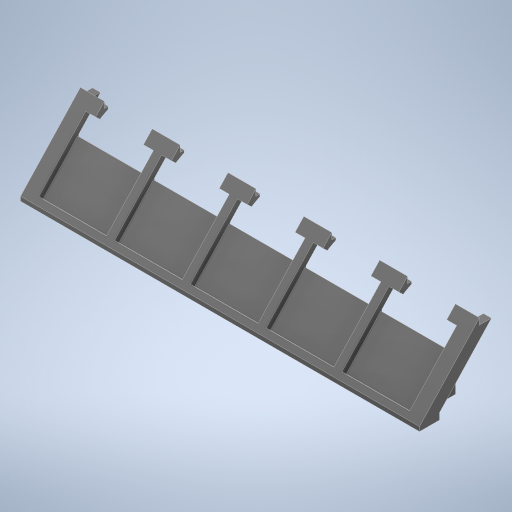
# Autodesk Inventor part: Front
Saved by Autodesk Inventor 2023 (Build 270158000, 158)
## iProperties
Created: 2024-03-20
Part Number: Front
Material: Generic
Document SubType Name: Modeling
Designer: noname
Density: 1 g/cm^3
Appearance: Smooth - Black
Author: noname
Autodesk Inventor part; units mm, degrees
ref_plane "YZ Plane" through (0, 0, 0) normal (1, 0, 0) x (0, 1, 0)
ref_plane "XZ Plane" through (0, 0, 0) normal (0, 1, 0) x (-1, 0, 0)
ref_plane "XY Plane" through (0, 0, 0) normal (0, 0, 1) x (1, 0, 0)
sketch "Sketch1" plane through (0, 0, 0) normal (1, 0, 0) x (0, 1, 0)
  line L0 (0, 0) -> (17.2, -16)
  line L1 (17.2, -16) -> (15.6, -16)
  line L2 (15.6, -16) -> (15.6, -19)
  line L3 (15.6, -19) -> (13.6298, -19)
  line L4 (13.6298, -19) -> (13.6298, -18.142)
  line L5 (1.6, -6) -> (0, -6)
  line L6 (0, -6) -> (0, 0)
  line L7 (1.6, -6) -> (1.6, -6.9515)
  line L8 (1.6, -6.9515) -> (13.6298, -18.142)
  dimension "d0" = 1.6
  dimension "d1" = 1.9702
  dimension "d3" = 14
  dimension "d4" = 4
  dimension "d7" = 6
  dimension "d8" = 3
  dimension "d10" = 10
  dimension "d13" = 1.6
  constraints: 18 end point, 3 perpendicular, 2 parallel, 1 horizontal, 1 vertical
  measures "d0" distance between parallel lines of L6 L7
  measures "d1" distance between parallel lines of L4 L2
  measures "d3" distance between parallel lines of L7 L2
  measures "d4" distance between parallel lines of L8 L0
  measures "d7" distance of L5.end L0.start
  measures "d8" distance between parallel lines of L1 L3
  measures "d10" distance between parallel lines of L1 L5
  measures "d13" distance of L0.end L1.end
extrude "Extrusion1" add sketch "Sketch1" along normal blind 100
ref_plane "Work Plane1" through (96.5, 0, 0) normal (1, 0, 0) x (0, 0, -1)
sketch "Sketch2" plane through (96.5, 0, 0) normal (1, 0, 0) x (0, 0, -1)
  line L0 (6.9515, 1.6) -> (18.142, 13.6298) projected
  line L1 (6, 1.6) -> (6.9515, 1.6) projected
  line L2 (6, 0) -> (6, 1.6) projected
  line L3 (0, 0) -> (6, 0) projected
  line L4 (16, 17.2) -> (0, 0) projected
  line L5 (16, 15.6) -> (16, 17.2) projected
  line L6 (19, 15.6) -> (16, 15.6) projected
  line L7 (19, 13.6298) -> (19, 15.6) projected
  line L8 (18.142, 13.6298) -> (19, 13.6298) projected
  line L9 (14.7401, 13.6433) -> (3.1416, 1.1749)
  line L10 (3.1416, 1.1749) -> (2.0433, 2.1966)
  line L11 (16.9367, 14.6) -> (19.0445, 14.6)
  arc A0 (16.9367, 14.6) -> (14.7401, 13.6433) centre (16.9367, 11.6) ccw
  point P0 (19, 14.6)
  dimension "d15" = 1.5
  dimension "d16" = 3
  dimension "d17" = 1
  dimension "d18" = 3
  constraints: 6 end point, 2 perpendicular, 2 point on circle, 2 point on line, 2 tangent, 1 centre point, 1 horizontal
  measures "d15" distance between parallel lines of L4 L9
  measures "d16" distance from line of point (0, 0) L10
  measures "d17" distance between parallel lines of L6 L11
  measures "d18" radius of A0
extrude "Extrusion2" cut sketch "Sketch2" against normal blind 17 contours L11 A0 L9 L10 L4 L5 L6 L7
sketch "Sketch3" plane through (79.5, 0, 0) normal (1, 0, 0) x (0, 0, -1)
  line L0 (2.0433, 2.1966) -> (16, 17.2) projected
  line L1 (3.1416, 1.1749) -> (2.0433, 2.1966) projected
  line L2 (14.7401, 13.6433) -> (3.1416, 1.1749) projected
  arc A0 (16.9367, 14.6) -> (14.7401, 13.6433) centre (16.9367, 11.6) ccw projected
  line L3 (19, 14.6) -> (16.9367, 14.6) projected
  line L4 (19, 15.6) -> (19, 14.6) projected
  line L5 (16, 15.6) -> (19, 15.6) projected
  line L6 (16, 17.2) -> (16, 15.6) projected
  line L7 (16, 17.2) -> (0, 0) projected
  line L8 (13.8264, 14.8634) -> (14.9337, 13.8334)
  dimension "d21" = 17.3
  constraints: 2 end point, 1 perpendicular, 1 point on circle, 1 point on line
  measures "d21" distance between parallel lines of L1 L8
extrude "Extrusion3" add sketch "Sketch3" along normal blind 2.5 contours L0 L6 L5 L4 L3 A0 L8
ref_plane "Work Plane2" through (88, 0, 0) normal (1, 0, 0) x (0, 0, -1)
mirror "Mirror1" about plane through (88, 0, 0) normal (1, 0, 0) of "Extrusion3"
pattern_linear "Rectangular Pattern1" count 5 spacing 19 along (-1, 0, 0) of "Extrusion3", "Mirror1", "Extrusion2"
sketch "Sketch5" plane through (100, 0, 0) normal (1, 0, 0) x (0, 0, -1)
  line L0 (6.9515, 1.6) -> (18.142, 13.6298) projected
  arc A0 (19, 15.5315) -> (12.0607, 7.0925) centre (20.0446, 7.6) ccw
  line L1 (3.1416, 1.1749) -> (14.7401, 13.6433) projected
  line L2 (14.7401, 13.6433) -> (3.1416, 1.1749) projected
  line L3 (19, 15.6) -> (16, 15.6) projected
  line L4 (6.9515, 1.6) -> (18.142, 13.6298) projected
  line L5 (18.142, 13.6298) -> (19, 13.6298) projected
  line L6 (19, 13.6298) -> (19, 15.6) projected
  line L7 (19, 15.6) -> (16, 15.6) projected
  line L8 (16, 15.6) -> (16, 17.2) projected
  line L9 (16, 17.2) -> (0, 0) projected
  line L10 (0, 0) -> (6, 0) projected
  line L11 (6, 0) -> (6, 1.6) projected
  line L12 (6, 1.6) -> (6.9515, 1.6) projected
  line L13 (11.812, 10.4956) -> (12.3978, 9.9507)
  line L14 (19, 14.6) -> (19, 15.6) projected
  line L15 (19, 15.6) -> (16, 15.6) projected
  line L16 (16, 15.6) -> (16, 17.2) projected
  line L17 (16, 17.2) -> (13.8264, 14.8634) projected
  line L18 (13.8264, 14.8634) -> (14.9337, 13.8334) projected
  arc A1 (16.9367, 14.6) -> (14.9337, 13.8334) centre (16.9367, 11.6) ccw projected
  line L19 (19, 14.6) -> (16.9367, 14.6) projected
  line L20 (14.9337, 13.8334) -> (14.9722, 13.7864)
  line L21 (19, 15.6) -> (16, 15.6) projected
  line L22 (17, 15.6) -> (17, 14.998)
  line L23 (14.7401, 13.6433) -> (14.9247, 13.8417)
  line L24 (13.8264, 14.8634) -> (14.9337, 13.8334) projected
  point P0 (14.1871, 13.0488)
  point P1 (11.812, 10.4956)
  point P2 (15.7777, 14.3671)
  dimension "d27" = 8
  dimension "d30" = 0.8
  dimension "d31" = 1
  constraints: 8 end point, 5 point on circle, 5 point on line, 3 perpendicular, 2 tangent, 1 centre point, 1 line through centre
  measures "d27" radius of A0
  measures "d30" distance of L13.start L13.end
  measures "d31" distance between parallel lines of L22 L16
extrude "Extrusion4" cut sketch "Sketch5" against normal through all contours A0 A1 L19 L6 L5 L0 | L13 L1 A0 | L1 L23 L18 L20 A0 | L19 A1 A0 L6 | L20 A1 A0 | A0 L22 L3 L6
sketch "Sketch6" plane through (100, 0, 0) normal (1, 0, 0) x (0, 0, -1)
  arc A0 (12.3978, 9.9507) -> (12.0607, 7.0925) centre (20.0446, 7.6) ccw projected
  line L0 (12.0607, 7.0925) -> (12.0607, 1.6)
  line L1 (6.9515, 1.6) -> (12.0607, 7.0925) projected
  line L2 (12.0607, 1.6) -> (6.9515, 1.6)
  point P0 (0, 0)
  constraints: 4 end point, 1 horizontal, 1 vertical
extrude "Extrusion5" add sketch "Sketch6" against normal up to surface (100 mm away)
sketch "Sketch7" plane through (100, 0, 0) normal (1, 0, 0) x (0, 0, -1)
  line L0 (6, 1.6) -> (12.0607, 1.6) projected
  line L1 (12.0446, 1.6) -> (12.0446, 10.2793)
  line L2 (12.3978, 9.9507) -> (11.812, 10.4956) projected
  arc A0 (12.3978, 9.9507) -> (12.0607, 7.0925) centre (20.0446, 7.6) ccw projected
  arc A1 (12.3978, 9.9507) -> (12.0607, 7.0925) centre (20.0446, 7.6) ccw projected
  line L3 (12.3978, 9.9507) -> (11.812, 10.4956) projected
  line L4 (11.812, 10.4956) -> (14.9247, 13.8417) projected
  line L5 (14.9247, 13.8417) -> (14.9337, 13.8334) projected
  arc A2 (15.7777, 14.3671) -> (14.9337, 13.8334) centre (16.9367, 11.6) ccw projected
  arc A3 (17, 14.998) -> (15.7777, 14.3671) centre (20.0446, 7.6) ccw projected
  line L6 (17, 14.998) -> (17, 15.6) projected
  line L7 (17, 15.6) -> (16, 15.6) projected
  line L8 (16, 15.6) -> (16, 17.2) projected
  line L9 (16, 17.2) -> (0, 0) projected
  line L10 (0, 0) -> (6, 0) projected
  line L11 (6, 0) -> (6, 1.6) projected
  line L12 (6, 1.6) -> (12.0607, 1.6) projected
  line L13 (12.0607, 1.6) -> (12.0607, 7.0925) projected
  constraints: 2 end point, 2 point on line, 1 tangent, 1 vertical
extrude "Extrusion6" cut sketch "Sketch7" against normal through all contours L11 L10 L9 L8 L7 L6 A3 A2 L5 L4 L2 L1 L0 keep common part
chamfer "Chamfer1" distance 0.31 angle 45 6 edges at (98.25, 10.4956, -11.812) (78.5, 10.4956, -11.812) (59.5, 10.4956, -11.812) (40.5, 10.4956, -11.812) (21.5, 10.4956, -11.812) (1.75, 10.4956, -11.812)
sketch "Sketch8" plane through (100, 0, 0) normal (1, 0, 0) x (0, 0, -1)
  line L0 (6, 0) -> (6, 1.6) projected
  line L1 (6, 1.6) -> (12.0446, 8.0979)
  line L2 (16, 17.2) -> (0, 0) projected
  line L3 (12.0446, 10.2793) -> (12.0446, 1.6) projected
  line L4 (12.0446, 10.2793) -> (12.0446, 1.6) projected
  line L5 (12.0446, 10.2793) -> (12.039, 10.2845) projected
  line L6 (12.0232, 10.7226) -> (12.039, 10.2845) projected
  line L7 (12.0232, 10.7226) -> (14.9247, 13.8417) projected
  line L8 (14.9247, 13.8417) -> (14.9337, 13.8334) projected
  arc A0 (15.7777, 14.3671) -> (14.9337, 13.8334) centre (16.9367, 11.6) ccw projected
  arc A1 (17, 14.998) -> (15.7777, 14.3671) centre (20.0446, 7.6) ccw projected
  line L9 (17, 14.998) -> (17, 15.6) projected
  line L10 (17, 15.6) -> (16, 15.6) projected
  line L11 (16, 15.6) -> (16, 17.2) projected
  line L12 (16, 17.2) -> (0, 0) projected
  line L13 (0, 0) -> (6, 0) projected
  line L14 (6, 0) -> (6, 1.6) projected
  line L15 (6, 1.6) -> (12.0446, 1.6) projected
  constraints: 2 end point, 1 parallel, 1 point on line
extrude "Extrusion7" cut sketch "Sketch8" against normal blind 2 contours L1 L3 L15
sketch "Sketch9" plane through (100, 0, 0) normal (1, 0, 0) x (0, 0, -1)
  line L0 (6, 1.6) -> (12.0446, 8.0979) projected
  line L1 (12.0446, 8.0979) -> (19.0233, 15.6)
  line L2 (17, 15.6) -> (17, 14.998) projected
  line L3 (19.0233, 15.6) -> (17, 15.6)
  line L4 (6, 1.6) -> (12.0446, 8.0979) projected
  line L5 (12.0446, 10.2793) -> (12.0446, 8.0979) projected
  line L6 (12.0446, 10.2793) -> (12.039, 10.2845) projected
  line L7 (12.0232, 10.7226) -> (12.039, 10.2845) projected
  line L8 (12.0232, 10.7226) -> (14.9247, 13.8417) projected
  line L9 (14.9247, 13.8417) -> (14.9337, 13.8334) projected
  arc A0 (15.7777, 14.3671) -> (14.9337, 13.8334) centre (16.9367, 11.6) ccw projected
  arc A1 (17, 14.998) -> (15.7777, 14.3671) centre (20.0446, 7.6) ccw projected
  line L10 (17, 14.998) -> (17, 15.6) projected
  line L11 (17, 15.6) -> (16, 15.6) projected
  line L12 (16, 15.6) -> (16, 17.2) projected
  line L13 (16, 17.2) -> (0, 0) projected
  line L14 (0, 0) -> (6, 0) projected
  line L15 (6, 0) -> (6, 1.6) projected
  constraints: 4 end point, 1 collinear, 1 perpendicular
extrude "Extrusion8" add sketch "Sketch9" against normal blind 2 contours L5 L6 L7 L8 L9 A0 A1 L2 L3 L1
ref_plane "Work Plane3" through (50, 0, 0) normal (-1, 0, 0) x (0, 0, 1)
mirror "Mirror2" about plane through (50, 0, 0) normal (-1, 0, 0) of "Extrusion7", "Extrusion8"
sketch "Sketch10" plane through (0, 0, -6) normal (0, -1, 0) x (1, 0, 0)
  line L0 (100, -10) -> (100, 6) projected
  line L1 (0, 6) -> (100, 6)
  line L2 (100, 6) -> (100, 5)
  line L3 (100, 5) -> (0, 5)
  line L4 (0, 5) -> (0, 6)
  dimension "d43" = 1
  constraints: 8 end point, 2 parallel, 1 horizontal, 1 perpendicular, 1 point on line
  measures "d43" distance between parallel lines of L1 L3
extrude "Extrusion9" cut sketch "Sketch10" against normal through all
body "Solid1"
